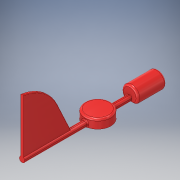
# Autodesk Inventor part: Direccion
Saved by Autodesk Inventor 2019 (Build 230136000, 136)
## iProperties
Created: 2019-12-17
Part Number: Direccion
Material: Generic
Document SubType Name: Modeling
Designer: Sergio
Density: 1 g/cm^3
Appearance: Light Red
Author: Sergio
Autodesk Inventor part; units mm, degrees
ref_plane "YZ Plane" through (0, 0, 0) normal (1, 0, 0) x (0, 1, 0)
ref_plane "XZ Plane" through (0, 0, 0) normal (0, 1, 0) x (-1, 0, 0)
ref_plane "XY Plane" through (0, 0, 0) normal (0, 0, 1) x (1, 0, 0)
sketch "Sketch1" plane through (0, 0, 0) normal (0, 1, 0) x (-1, 0, 0)
  line L0 (-4, -107.5) -> (4, -107.5)
  line L1 (4, 107.5) -> (-4, 107.5)
  line L2 (-4, -107.5) -> (4, 107.5) construction
  line L3 (4, -107.5) -> (-4, 107.5) construction
  line L4 (-4, 107.5) -> (-4, 7.711939)
  line L5 (-4, -32.5) -> (-4, -107.5)
  line L6 (4, -107.5) -> (4, -32.5)
  line L7 (4, 7.711939) -> (4, 107.5)
  arc A0 (4, -32.5) -> (4, 7.711939) centre (0, -12.394031) ccw
  arc A1 (-4, 7.711939) -> (-4, -32.5) centre (0, -12.394031) ccw
  point P0 (0, 0)
  dimension "d0" = 8
  dimension "d1" = 215
  dimension "d14" = 20.5
  dimension "d15" = 20.5
  dimension "d16" = 8
  dimension "d17" = 75
  constraints: 16 end point, 7 parallel, 4 point on circle, 2 centre point, 2 midpoint, 2 perpendicular, 1 horizontal
  measures "d0" distance of L1.end L1.start
  measures "d1" distance of L1.start L0.end
  measures "d14" radius of A0
  measures "d15" radius of A1
  measures "d16" distance between parallel lines of L5 L6
  measures "d17" distance of L5.start L0.start
extrude "Extrusion1" add sketch "Sketch1" along normal blind 8
sketch "Sketch2" plane through (0, 0, 0) normal (1, 0, 0) x (0, 1, 0)
  line L0 (8, 107.5) -> (8, 32.5)
  line L1 (8, 32.5) -> (53.235766, 53.593784)
  line L2 (8, 107.5) -> (93, 107.5)
  arc A0 (53.235766, 53.593784) -> (93, 107.5) centre (23.652487, 117.035329) ccw
  point P0 (0, 0)
  dimension "d6" = 75
  dimension "d7" = 85
  dimension "d9" = 65
  dimension "d11" = 70
  constraints: 6 end point, 2 point on circle, 1 centre point, 1 horizontal, 1 tangent
  measures "d6" distance of L0.start L0.end
  measures "d7" distance of L0.start L2.end
  measures "d9" angle of L0 L1
  measures "d11" radius of A0
extrude "Extrusion2" add sketch "Sketch2" along normal mid plane 4
sketch "Sketch4" plane through (4, 0, -107.5) normal (0, 0, -1) x (-1, 0, 0)
  arc A0 (13.746951, 0) -> (-6.746951, 0) centre (3.5, 8) ccw
  line L0 (0, 8) -> (8, 8)
  line L1 (8, 0) -> (8, 8)
  line L2 (-6.746951, 0) -> (13.746951, 0)
  line L3 (0, 0) -> (-16.5, 0)
  point P0 (4, 0)
  point P1 (0, 0)
  dimension "d19" = 26
  dimension "d20" = 0
  dimension "d21" = 4.5
  dimension "d76" = 0
  constraints: 2 end point, 2 point on circle, 1 centre point, 1 horizontal
  measures "d19" diameter of A0
  measures "d20" distance from line of L0 A0.centre
  measures "d21" distance from line of L1 A0.centre
  measures "d76" distance between parallel lines of L3 L2
extrude "Extrusion3" add sketch "Sketch4" against normal blind 45
fillet "Fillet2" radius 0.8 2 edges at (-2, 79.9845, 75.4817) (-2, 30.6179, 43.0469)
fillet "Fillet3" radius 0.8 2 edges at (2, 79.9845, 75.4817) (2, 30.6179, 43.0469)
fillet "Fillet14" radius 3 8 edges at (4, 8, 57.606) (-4, 8, 57.606) (4, 8, -47.5) (-4, 8, -47.5) (-4, 0, 57.606) (4, 0, 57.606) (-4, 0, -47.5) (4, 0, -47.5)
sketch "Sketch15" plane through (0, 8, 0) normal (0, 1, 0) x (1, 0, 0)
  circle A0 centre (0, 12.394031) radius 20.5
  arc A1 (-1, 32.869626) -> (-1, -8.081564) centre (0, 12.394031) ccw
  constraints: 2 concentric, 1 centre point
extrude "Extrusion9" add sketch "Sketch15" along normal blind 6
sketch "Sketch16" plane through (0, 0, 0) normal (0, -1, 0) x (1, 0, 0)
  circle A0 centre (0, -12.394031) radius 12.4
  arc A1 (1, -32.869626) -> (1, 8.081564) centre (0, -12.394031) ccw
  point P0 (0, 0)
  dimension "d79" = 24.8
  constraints: 1 centre point, 1 concentric
  measures "d79" diameter of A0
extrude "Extrusion10" cut sketch "Sketch16" against normal blind 9
sketch "Sketch17" plane through (0, 9, -12.394031) normal (0, -1, 0) x (1, 0, 0)
  circle A0 centre (0, 0) radius 8
  point P0 (0, 12.394031)
  dimension "d82" = 16
  constraints: 1 centre point
  measures "d82" diameter of A0
extrude "Extrusion11" cut sketch "Sketch17" against normal blind 2
fillet "Fillet18" radius 3 1 edges at (-20.5, 14, -12.394)
fillet "Fillet19" radius 3 2 edges at (0.5, 21, -62.5) (0.5, 21, -107.5)
fillet "Fillet20" radius 2 7 edges at (-3.276, 6.9545, 7.8425) (-4, 4, 7.7119) (-3.2765, 1.0461, 7.8424) (3.276, 6.9545, 7.8425) (4, 4, 7.7119) (3.2765, 1.0461, 7.8424) (0, 8, 8.106)
fillet "Fillet21" radius 2 7 edges at (4, 4, -32.5) (3.2765, 1.0461, -32.6305) (0, 8, -32.894) (-3.2633, 6.9692, -32.6326) (-4, 4, -32.5) (-3.2759, 1.0455, -32.6306) (3.276, 6.9545, -32.6306)
fillet "Fillet22" radius 1.5 1 edges at (-8, 11, -12.394)
fillet "Fillet23" radius 0.5 1 edges at (-8, 9, -12.394)
body "Solid1"
